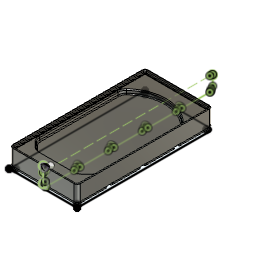
Gridfinity-RyobiBatteryHolder_v3 (Autodesk Fusion 360 design; units mm, degrees)
Autodesk Fusion 360 part; units mm, degrees
note: some values were not read from the file. Chosen so that the rebuilt part matches the saved one: which bodies a step acts on. Set by a fixed rule: which sketch regions a step uses; which face or edge a step refers to.
sketch "BaseUnit" plane through (0, 0, 0) normal (0, 0, 1) x (1, 0, 0)
  line L0 (42, 42) -> (0, 42)
  line L1 (0, 42) -> (0, 0)
  line L2 (0, 0) -> (42, 0)
  line L3 (42, 0) -> (42, 42)
  line L4 (42, 42) -> (0, 0) construction
  line L5 (0, 42) -> (42, 0) construction
  circle A0 centre (10.95, 31.05) radius 3.25
  circle A1 centre (10.95, 31.05) radius 1.5
  line L6 (2.15, 2.15) -> (39.85, 2.15)
  line L7 (39.85, 2.15) -> (39.85, 39.85)
  line L8 (39.85, 39.85) -> (2.15, 39.85)
  line L9 (2.15, 39.85) -> (2.15, 2.15)
  line L10 (2.95, 2.95) -> (39.05, 2.95)
  line L11 (39.05, 2.95) -> (39.05, 39.05)
  line L12 (39.05, 39.05) -> (2.95, 39.05)
  line L13 (2.95, 39.05) -> (2.95, 2.95)
  line L14 (0, 2.5) -> (0, 20) construction
  line L15 (20, 0) -> (2.5, 0) construction
  line L16 (21, 21) -> (21, 42) construction
  line L17 (21, 21) -> (42, 21) construction
  circle A2 centre (31.05, 31.05) radius 3.25
  circle A3 centre (31.05, 31.05) radius 1.5
  circle A4 centre (10.95, 10.95) radius 3.25
  circle A5 centre (10.95, 10.95) radius 1.5
  circle A6 centre (31.05, 10.95) radius 3.25
  circle A7 centre (31.05, 10.95) radius 1.5
  dimension "d3" = 42
  dimension "d4" = 42
  dimension "d5" = 6.5
  dimension "d6" = 3
  dimension "d11" = -2.15
  dimension "d12" = -2.95
  dimension "d13" = 8
  dimension "d14" = 8
  constraint horizontal L0
  constraint perpendicular L0 L1
  constraint parallel L0 L2
  constraint parallel L1 L3
  constraint concentric A0 A1
  constraint coincident L1.end L2.start
  constraint midpoint L5 L16.start
  constraint midpoint L0 L16.end
  constraint midpoint L3 L17.end
  constraint symmetric A0 L16 A2
  constraint symmetric A1 L16 A3
  constraint symmetric A0 L17 A4
  constraint symmetric A1 L17 A5
  constraint symmetric L17 A2 A6
  constraint symmetric L17 A3 A7
  measures "d3" distance of L1.end L2.end
  measures "d4" distance of L0.end L1.end
  measures "d5" diameter of A0
  measures "d6" diameter of A1
  measures "d13" distance of A0.centre L12
  measures "d14" distance of A0.centre L13
extrude "Extrude1" add sketch "BaseUnit" along normal blind 5 contours L0 L1 L2 L3 | A0 | A1 | L6 L7 L8 L9 | L10 L11 L12 L13 | A2 | A3 | A4 | A5 | A6 | A7 makes body 1
ref_plane "WorkPlane1" through (21, 21, 2.5) normal (0, -1, 0) x (1, 0, 0)
sketch "CuttingProfile" plane through (0, 21, 0) normal (0, -1, 0) x (1, 0, 0)
  line L0 (0, 0) -> (41.5, 0) construction
  line L1 (41.5, 0) -> (41.5, -4.75) construction
  line L2 (41.5, -4.75) -> (0, -4.75) construction
  line L3 (0, -4.75) -> (0, 0)
  line L4 (0, -4.75) -> (1.8, -4.75) construction
  line L5 (2.7302, 0) -> (0, 0)
  line L6 (0, -4.75) -> (-3.4297, -4.75)
  line L7 (42, 0) -> (0, 0) construction
  line L8 (0, 0) -> (0, 5) construction
  line L9 (0, 5) -> (42, 5) construction
  line L10 (42, 5) -> (42, 0) construction
  line L11 (0, 5) -> (2.4, 2.6)
  line L12 (0, 5) -> (1.9526, 5) construction
  line L13 (2.4, 2.6) -> (2.4, 0.8)
  line L14 (2.4, 0.8) -> (3.2, 0)
  line L15 (2.4, 0.8) -> (2.7859, 0.8) construction
  line L16 (0, 5) -> (-10, 5)
  line L17 (-10, 5) -> (-10, 0)
  line L18 (3.2, 0) -> (-10, 0)
  line L19 (2.4, 21.8) -> (3.2, 21)
  line L20 (0, 26) -> (2.4, 23.6)
  line L21 (2.4, 23.6) -> (2.4, 21.8)
  line L22 (0, 26) -> (-10, 26)
  line L23 (-10, 26) -> (-10, 21)
  line L24 (-10, 21) -> (3.2, 21)
  line L25 (-0.1768, 25.8232) -> (2.15, 23.4964)
  line L26 (2.15, 23.4964) -> (2.15, 21.6964)
  line L27 (2.15, 21.6964) -> (3.0232, 20.8232)
  line L28 (1.91, 23.7364) -> (-1.0539, 26.7004)
  line L29 (0, 26) -> (0, 21)
  dimension "d58" = 45
  dimension "d60" = 1.8
  dimension "d61" = 45
  dimension "d70" = 2.4
  dimension "d80" = 5
  dimension "d91" = 1.8
  dimension "d92" = 2.4
  dimension "d94" = 45
  dimension "d95" = 45
  dimension "d96" = 5
  dimension "d97" = 21
  dimension "d98" = 10
  dimension "d99" = 10
  dimension "d100" = 0.25
  constraint horizontal L4
  constraint coincident L2.end L3.start
  constraint coincident L0.start L3.end
  constraint perpendicular L3 L6
  constraint horizontal L12
  constraint coincident L8.end L9.start
  constraint vertical L13
  constraint horizontal L15
  constraint perpendicular L8 L16
  constraint perpendicular L16 L17
  constraint perpendicular L17 L18
  constraint coincident L0 L14.end
  constraint coincident L5.start L18
  constraint vertical L21
  constraint vertical L0.start L20.start
  constraint horizontal L22
  constraint perpendicular L22 L23
  constraint vertical L14.end L19.end
  constraint coincident L25 L28.start
  constraint parallel L25 L28
  constraint coincident L24 L29.end
  constraint perpendicular L24 L29
  measures "d58" angle of L11 L12
  measures "d60" distance of L11.end L13.end
  measures "d61" angle of L14 L15
  measures "d70" horizontal distance of L8.end L11.end
  measures "d80" distance of L16.end L17.end
  measures "d91" distance of L19.start L20.end
  measures "d92" horizontal distance of L20.start L20.end
  measures "d94" angle of L8 L20
  measures "d95" angle of L8 L19
  measures "d96" distance of L22.end L23.end
  measures "d97" distance of L0 L19.end
  measures "d98" distance of L8 L17
  measures "d99" distance of L8 L23
sketch "fillietSketch" plane through (0, 0, 5) normal (0, 0, 1) x (-1, 0, 0)
  line L0 (-42, 0) -> (-42, -42) construction
  line L1 (-42, -42) -> (0, -42) construction
  line L2 (0, -42) -> (0, 0) construction
  line L3 (0, 0) -> (-42, 0) construction
  line L4 (-4, -42) -> (-38, -42)
  line L5 (-42, -38) -> (-42, -4)
  line L6 (-38, 0) -> (-4, 0)
  line L7 (0, -4) -> (0, -38)
  arc A0 (-4, -42) -> (0, -38) centre (-4, -38) ccw
  arc A1 (-42, -38) -> (-38, -42) centre (-38, -38) ccw
  arc A2 (-38, 0) -> (-42, -4) centre (-38, -4) ccw
  arc A3 (0, -4) -> (-4, 0) centre (-4, -4) ccw
  dimension "d51" = 4
  constraint horizontal L4
  constraint vertical L5
  constraint horizontal L6
  constraint vertical L7
  constraint tangent L4 A0
  constraint tangent L7 A0
  constraint tangent L4 A1
  constraint tangent L5 A1
  constraint equal A0 A1
  constraint tangent L5 A2
  constraint tangent L6 A2
  constraint equal A0 A2
  constraint tangent L6 A3
  constraint tangent L7 A3
  constraint equal A0 A3
  constraint collinear L1 L4
  constraint collinear L3 L6
  constraint collinear L0 L5
  constraint collinear L2 L7
  measures "d51" radius of A0
sweep "Sweep1" cut profiles "CuttingProfile" path "fillietSketch" along L6 A2 L5 A1 L4 A0 L7 A3 section 1 contours L5 L11 L13 L14 L16 L17 L18 bodies 1
extrude "Extrude6" cut sketch "BaseUnit" along normal through all contours A1 | A3 | A5 | A7 bodies 1
extrude "Extrude7" cut sketch "BaseUnit" along normal blind 4 contours A0 | A2 | A4 | A6 bodies 1
chamfer "Chamfer2" distance 1.7 angle 45 4 edges at (7.9199, 9.7747, 4) (28.0199, 9.7747, 4) (7.9199, 29.8747, 4) (28.0199, 29.8747, 4) on bodies 1
pattern_linear "R-Pattern2" count 4 spacing 42 along (0, 1, 0) count 2 spacing 42 along (1, 0, 0) of bodies 1 makes body 2 at (23.9835, 59.9901, 5) makes body 3 at (23.9835, 101.9901, 5) makes body 4 at (65.9835, 17.9901, 5) makes body 5 at (65.9835, 59.9901, 5) makes body 6 at (65.9835, 101.9901, 5) makes body 7 at (23.9835, 143.9901, 5) makes body 8 at (65.9835, 143.9901, 5)
sketch "filletSketchFullUnit" plane through (0, 0, 0) normal (0, 0, 1) x (1, 0, 0)
  line L0 (4, 0) -> (80, 0)
  line L1 (84, 4) -> (84, 164)
  line L2 (80, 168) -> (4, 168)
  line L3 (0, 164) -> (0, 4)
  arc A0 (4, 168) -> (0, 164) centre (4, 164) ccw
  arc A1 (0, 4) -> (4, 0) centre (4, 4) ccw
  arc A2 (80, 0) -> (84, 4) centre (80, 4) ccw
  arc A3 (84, 164) -> (80, 168) centre (80, 164) ccw
  line L4 (83.75, 4) -> (83.75, 164)
  arc A4 (83.75, 164) -> (80, 167.75) centre (80, 164) ccw
  line L5 (80, 167.75) -> (4, 167.75)
  arc A5 (4, 167.75) -> (0.25, 164) centre (4, 164) ccw
  line L6 (0.25, 164) -> (0.25, 4)
  arc A6 (0.25, 4) -> (4, 0.25) centre (4, 4) ccw
  line L7 (4, 0.25) -> (80, 0.25)
  arc A7 (80, 0.25) -> (83.75, 4) centre (80, 4) ccw
  point P0 (84, 0)
  point P1 (0, 168)
  dimension "d82" = 84
  dimension "d83" = 168
  dimension "d84" = 4
  dimension "d123" = -0.25
  constraint horizontal L0
  constraint vertical L1
  constraint horizontal L2
  constraint vertical L3
  constraint coincident P1 L2
  constraint coincident P1 L3
  constraint tangent L2 A0
  constraint tangent L3 A0
  constraint coincident origin L0
  constraint coincident origin L3
  constraint tangent L0 A1
  constraint tangent L3 A1
  constraint equal A0 A1
  constraint coincident P0 L0
  constraint coincident P0 L1
  constraint tangent L0 A2
  constraint tangent L1 A2
  constraint equal A0 A2
  constraint tangent L2 A3
  constraint tangent L1 A3
  constraint equal A0 A3
  measures "d82" distance of origin P0
  measures "d83" distance of origin P1
  measures "d84" radius of A0
extrude "Extrude8" add sketch "filletSketchFullUnit" along normal blind 16 from surface at 5 contours L0 L1 L2 L3 A0 A1 A2 A3 | L4 A4 L5 A5 L6 A6 L7 A7 bodies 1 7 8 2 3 4 5 6
sweep "Sweep2" add profiles "CuttingProfile" path "filletSketchFullUnit" along L0 A2 L1 A3 L2 A0 L3 A1 section 1 contours L24 L25 L26 L27 L28 L29 bodies 1
extrude "Extrude10" cut sketch "filletSketchFullUnit" along normal blind 100 bodies 1
ref_plane "WorkPlane3" through (42, 84, 15.0732) normal (1, 0, 0) x (0, 1, 0)
sketch "TopLipFilet" plane through (42, 0, 0) normal (1, 0, 0) x (0, 1, 0)
  line L0 (0.25, 4.75) -> (0.25, 25.3964)
  line L1 (0.25, 25.3964) -> (0.25, 4.75)
  line L2 (0.25, 5) -> (0.25, 4.75)
  line L3 (0.25, 4.75) -> (0.25, 5)
  line L4 (0.25, 4.75) -> (0.25, 25.3964)
  arc A0 (1.2743, 24.3722) -> (0.25, 23.9479) centre (0.85, 23.9479) ccw
  line L5 (0.25, 4.75) -> (0.25, 25.3964)
  line L6 (167.75, 4.75) -> (167.75, 25.3964)
  line L7 (123.6, 2.6) -> (126, 5)
  line L8 (123.6, 0.8) -> (123.6, 2.6)
  line L9 (122.8, 0) -> (123.6, 0.8)
  line L10 (122, 0) -> (122.8, 0)
  line L11 (86.4, 2.6) -> (84, 5)
  line L12 (86.4, 0.8) -> (86.4, 2.6)
  line L13 (87.2, 0) -> (86.4, 0.8)
  line L14 (87.2, 0) -> (88, 0)
  line L15 (88, 0) -> (122, 0)
  line L16 (165.6, 2.6) -> (167.75, 4.75)
  line L17 (165.6, 0.8) -> (165.6, 2.6)
  line L18 (164.8, 0) -> (165.6, 0.8)
  line L19 (164, 0) -> (164.8, 0)
  line L20 (128.4, 2.6) -> (126, 5)
  line L21 (128.4, 0.8) -> (128.4, 2.6)
  line L22 (129.2, 0) -> (128.4, 0.8)
  line L23 (129.2, 0) -> (130, 0)
  line L24 (130, 0) -> (164, 0)
  line L25 (81.6, 2.6) -> (84, 5)
  line L26 (81.6, 0.8) -> (81.6, 2.6)
  line L27 (80.8, 0) -> (81.6, 0.8)
  line L28 (80, 0) -> (80.8, 0)
  line L29 (44.4, 2.6) -> (42, 5)
  line L30 (44.4, 0.8) -> (44.4, 2.6)
  line L31 (45.2, 0) -> (44.4, 0.8)
  line L32 (45.2, 0) -> (46, 0)
  line L33 (46, 0) -> (80, 0)
  line L34 (39.6, 2.6) -> (42, 5)
  line L35 (39.6, 0.8) -> (39.6, 2.6)
  line L36 (38.8, 0) -> (39.6, 0.8)
  line L37 (38, 0) -> (38.8, 0)
  line L38 (2.4, 2.6) -> (0.25, 4.75)
  line L39 (2.4, 0.8) -> (2.4, 2.6)
  line L40 (3.2, 0) -> (2.4, 0.8)
  line L41 (3.2, 0) -> (4, 0)
  line L42 (4, 0) -> (38, 0)
  line L43 (0.25, 25.3964) -> (1.2743, 24.3722)
  line L44 (164, 25.3964) -> (4, 25.3964)
  line L45 (4, 25.3964) -> (0.25, 25.3964)
  line L46 (167.75, 25.3964) -> (164, 25.3964)
  dimension "d132" = 1.2
  dimension "d141" = 45
  constraint tangent L0 A0
  constraint coincident L0 A0.end
  constraint tangent A0 L43
  measures "d132" diameter of A0
  measures "d141" angle of L5 L43
sweep "Sweep4" cut profiles "TopLipFilet" path "filletSketchFullUnit" along A4 L5 A5 L6 A6 L7 A7 L4 section 1 contours L0 L1 L4 A0 L5 L43 bodies 1
extrude "Extrude9" cut 1 faces at (28.9488, 110.6667, 21) along direction (0, 0, -1) up to surface (14.8 mm away) on bodies 1 bodies 1
ref_plane "WorkPlane2" through (42, 84, 13.6) normal (1, 0, 0) x (0, -1, 0)
sketch "Sketch11" plane through (42, 0, 0) normal (1, 0, 0) x (0, 1, 0)
  arc A0 (0.85, 17.5479) -> (0.25, 16.9479) centre (0.85, 16.9479) ccw
  arc A1 (209.75, 16.9479) -> (209.15, 17.5479) centre (209.15, 16.9479) ccw
  line L0 (0.25, 4.75) -> (0.25, 16.9479)
  line L1 (209.75, 4.75) -> (209.75, 16.9479)
  line L2 (207.6, 2.6) -> (209.75, 4.75)
  line L3 (123.6, 2.6) -> (126, 5)
  line L4 (123.6, 0.8) -> (123.6, 2.6)
  line L5 (122.8, 0) -> (123.6, 0.8)
  line L6 (122, 0) -> (122.8, 0)
  line L7 (86.4, 2.6) -> (84, 5)
  line L8 (86.4, 0.8) -> (86.4, 2.6)
  line L9 (87.2, 0) -> (86.4, 0.8)
  line L10 (87.2, 0) -> (88, 0)
  line L11 (88, 0) -> (122, 0)
  line L12 (207.6, 0.8) -> (207.6, 2.6)
  line L13 (206.8, 0) -> (207.6, 0.8)
  line L14 (206, 0) -> (206.8, 0)
  line L15 (170.4, 2.6) -> (168, 5)
  line L16 (170.4, 0.8) -> (170.4, 2.6)
  line L17 (171.2, 0) -> (170.4, 0.8)
  line L18 (171.2, 0) -> (172, 0)
  line L19 (172, 0) -> (206, 0)
  line L20 (165.6, 2.6) -> (168, 5)
  line L21 (165.6, 0.8) -> (165.6, 2.6)
  line L22 (164.8, 0) -> (165.6, 0.8)
  line L23 (164, 0) -> (164.8, 0)
  line L24 (128.4, 2.6) -> (126, 5)
  line L25 (128.4, 0.8) -> (128.4, 2.6)
  line L26 (129.2, 0) -> (128.4, 0.8)
  line L27 (129.2, 0) -> (130, 0)
  line L28 (130, 0) -> (164, 0)
  line L29 (81.6, 2.6) -> (84, 5)
  line L30 (81.6, 0.8) -> (81.6, 2.6)
  line L31 (80.8, 0) -> (81.6, 0.8)
  line L32 (80, 0) -> (80.8, 0)
  line L33 (44.4, 2.6) -> (42, 5)
  line L34 (44.4, 0.8) -> (44.4, 2.6)
  line L35 (45.2, 0) -> (44.4, 0.8)
  line L36 (45.2, 0) -> (46, 0)
  line L37 (46, 0) -> (80, 0)
  line L38 (39.6, 2.6) -> (42, 5)
  line L39 (39.6, 0.8) -> (39.6, 2.6)
  line L40 (38.8, 0) -> (39.6, 0.8)
  line L41 (38, 0) -> (38.8, 0)
  line L42 (2.4, 2.6) -> (0.25, 4.75)
  line L43 (2.4, 0.8) -> (2.4, 2.6)
  line L44 (3.2, 0) -> (2.4, 0.8)
  line L45 (3.2, 0) -> (4, 0)
  line L46 (4, 0) -> (38, 0)
  line L47 (4, 17.5479) -> (0.85, 17.5479) construction
  line L48 (206, 17.5479) -> (4, 17.5479) construction
  line L49 (209.15, 17.5479) -> (206, 17.5479)
  line L50 (2.8464, 21) -> (2.8464, 17.5479)
  line L51 (2.8464, 19.8) -> (1.45, 18.4036)
  line L52 (2.8464, 19.8) -> (9.0539, 19.8) construction
  line L53 (1.45, 6.2) -> (1.45, 18.4036)
  line L54 (2.8464, 6.2) -> (2.8464, 22)
  line L55 (2.8464, 6.2) -> (1.45, 6.2)
  point P0 (2.8464, 21)
  point P1 (2.8464, 6.2)
  dimension "d144" = 1.2
  dimension "d148" = 45
  dimension "d159" = 1.9749
  constraint vertical L50
  constraint coincident P0 L50.start
  constraint horizontal L52
  constraint parallel L0 L53
  constraint coincident L51.start L50
  constraint coincident L47 L50.end
  constraint coincident P1 L54.start
  constraint coincident L50 L54.end
  constraint perpendicular L54 L55
  measures "d144" distance of P0 L51.start
  measures "d148" angle of L51 L53
  measures "d159" distance of L51.start L51.end
sketch "CuttingProfileInternal" plane through (42, 0, 0) normal (1, 0, 0) x (0, 1, 0)
  line L0 (0, 5) -> (0, 24.1979)
  line L1 (2.8464, 21) -> (2.8464, 6.2)
  line L2 (2.8464, 19.8) -> (1.45, 18.4036)
  line L3 (2.8464, 19.8) -> (2.0236, 19.8) construction
  line L4 (1.45, 18.4036) -> (1.45, 6.2)
  line L5 (2.8464, 6.2) -> (1.45, 6.2)
  line L6 (0.25, 4.75) -> (0.25, 23.9479)
  point P0 (2.8464, 21)
  dimension "d114" = 1.2
  dimension "d115" = 45
  dimension "d157" = 1.9749
  constraint vertical L1
  constraint horizontal L3
  constraint vertical L4
  constraint horizontal L5
  constraint coincident L1.end L5.start
  constraint vertical P0 L1.end
  constraint coincident L2.start L1
  constraint coincident P0 L1.start
  measures "d114" distance of P0 L2.start
  measures "d115" angle of L2 L3
  measures "d157" distance of L2.start L2.end
sweep "Sweep3" cut profiles "CuttingProfileInternal" path "filletSketchFullUnit" along L0 A2 L1 A3 L2 A0 L3 A1 section 1 bodies 1
move_face "OffsetFaces2" offset 9 1 faces at (55.5167, 57.3333, 6.2) on bodies 1
sketch "Sketch12" plane through (0, 0, 15.2) normal (0, 0, 1) x (-1, 0, 0)
  line L0 (-4.5, -134.0718) -> (-4.5, -16.9999)
  line L1 (-79.5, -134.0718) -> (-79.5, -16.9999)
  line L2 (-79.5, -16.9999) -> (-4.5, -16.9999)
  arc A0 (-79.5, -134.0718) -> (-4.5, -134.0718) centre (-42, -100.9999) ccw
  line L3 (-4.5, -29.0208) -> (-16.5208, -16.9999)
  line L4 (-67.4792, -16.9999) -> (-79.5, -29.0208)
  arc A1 (-80, -1.45) -> (-82.55, -4) centre (-80, -4) ccw
  line L5 (-82.55, -4) -> (-82.55, -164)
  arc A2 (-82.55, -164) -> (-80, -166.55) centre (-80, -164) ccw
  line L6 (-80, -166.55) -> (-4, -166.55)
  arc A3 (-4, -166.55) -> (-1.45, -164) centre (-4, -164) ccw
  line L7 (-1.45, -164) -> (-1.45, -4)
  arc A4 (-1.45, -4) -> (-4, -1.45) centre (-4, -4) ccw
  line L8 (-4, -1.45) -> (-80, -1.45)
  point P0 (-42, -16.9999)
  point P1 (-42, -2.8464)
  dimension "d162" = 75
  dimension "d163" = 100
  dimension "d164" = 45
  dimension "d165" = 45
  dimension "d166" = 134
  dimension "d167" = 17
  constraint vertical L0
  constraint vertical L1
  constraint perpendicular L0 L2
  constraint midpoint L2 P0
  constraint vertical A0.centre P0
  constraint coincident L0 L3.start
  constraint coincident L2 L3.end
  constraint coincident L2 L4.start
  constraint coincident L1 L4.end
  constraint equal L3 L4
  constraint vertical P0 P1
  measures "d162" distance of L0.end L1.end
  measures "d163" diameter of A0
  measures "d164" angle of L0 L3
  measures "d165" angle of L1 L4
  measures "d167" distance of L4.start L4.end
extrude "Extrude11" add sketch "Sketch12" along normal blind 5 contours L0 L2 L3 | L1 L2 L4 | A1 L5 A2 L6 A3 L7 A4 L8 bodies 1
fillet "Fillet7" radius 10 4 edges at (67.4792, 16.9999, 17.7) (79.5, 29.0208, 17.7) (16.5208, 16.9999, 17.7) (4.5, 29.0208, 17.7) on bodies 1
fillet "Fillet8" radius 10 2 edges at (79.5, 134.0718, 17.7) (4.5, 134.0718, 17.7) on bodies 1
chamfer "Chamfer3" distance 1 angle 45 12 edges at (42, 150.9999, 20.2) (78.6856, 134.0002, 20.2) (79.5, 81.6051, 20.2) (78.7388, 29.3361, 20.2) (73.4896, 23.0104, 20.2) (67.1639, 17.7612, 20.2) (42, 16.9999, 20.2) (16.8361, 17.7612, 20.2) (10.5104, 23.0104, 20.2) (5.2612, 29.3361, 20.2) (4.5, 81.6051, 20.2) (5.3144, 134.0002, 20.2) on bodies 1
fillet "Fillet9" radius 1 12 edges at (10.5104, 23.0104, 15.2) (16.8361, 17.7612, 15.2) (42, 16.9999, 15.2) (67.1639, 17.7612, 15.2) (73.4896, 23.0104, 15.2) (78.7388, 29.3361, 15.2) (79.5, 81.6051, 15.2) (78.6856, 134.0002, 15.2) (42, 150.9999, 15.2) (5.3144, 134.0002, 15.2) (4.5, 81.6051, 15.2) (5.2612, 29.3361, 15.2) on bodies 1
equation "GridsDeep = 4" comment "The number of grids deep for the unit"
equation "GridsWide = 2" comment "The Number of gridsWide The unit is"
equation "d3 = GridOuterSize"
equation "d4 = GridOuterSize"
equation "ToleranceMagnet = 0.05 mm"
equation "DiamteterMagnet = 6 mm"
equation "GridOuterSize = 42 mm"
equation "ChamferGridBase = 7.5 rad"
equation "d76 = GridsDeep"
equation "d77 = GridsWide"
equation "d78 = GridOuterSize"
equation "d79 = -GridOuterSize"
equation "StorageOffset = 0.25 mm"
equation "d82 = GridOuterSize * GridsWide"
equation "d83 = GridOuterSize * GridsDeep"
equation "NestingDepth = 5 mm"
equation "WallThickness = 1.2 mm"
equation "GridsHigh = 3 / 6"
equation "d89 = GridOuterSize * GridsHigh - NestingDepth"
equation "d96 = NestingDepth"
equation "d97 = GridOuterSize * GridsHigh - NestingDepth + 5 mm"
equation "d99 = d98"
equation "d112 = -WallThickness"
equation "VerticalDividerNumberOfSection = 3"
equation "d114 = WallThickness"
equation "d132 = WallThickness"
equation "d144 = WallThickness"
equation "d161 = 14 mm - 5 mm"
equation "d165 = d164"
named bodies: "Gridfinity-RyobiBatteryHolder", "StorageBlank (1)", "StorageBlank (3)"
